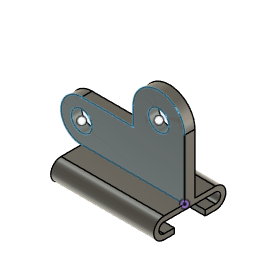
que6 v3 (Autodesk Fusion 360 design; units mm, degrees)
Autodesk Fusion 360 part; units mm, degrees
sketch "Sketch1" plane through (0, 0, 0) normal (0, 1, 0) x (1, 0, 0)
  line L0 (0, 0) -> (0, -58)
  line L1 (-50, -58) -> (-50, -40)
  line L2 (-50, -40) -> (-100, -40)
  line L3 (-100, 0) -> (0, 0)
  arc A0 (-50, -58) -> (0, -58) centre (-25, -58) ccw
  arc A1 (-100, 0) -> (-100, -40) centre (-100, -20) ccw
  circle A2 centre (-25, -58) radius 10
  circle A3 centre (-100, -20) radius 10
  dimension "d1" = 58
  dimension "d3" = 50
  dimension "d4" = 18
  dimension "d5" = 50
  dimension "d6" = 20
  dimension "d7" = 20
  constraint coincident L0.start L3.end
  constraint vertical L0
  constraint perpendicular L1 L2
  constraint concentric A0 A2
  constraint concentric A1 A3
  measures "d1" distance of L0.start L0.end
  measures "d3" distance of L0.end L1.start
  measures "d4" distance of L1.start L1.end
  measures "d5" distance of L1.end L2.end
  measures "d6" diameter of A2
  measures "d7" diameter of A3
extrude "Extrude1" add sketch "Sketch1" along normal blind 10
sketch "Sketch4" plane through (0, 0, 0) normal (1, 0, 0) x (0, 1, 0)
  line L0 (30, 0) -> (-20, 0)
  arc A0 (-20, 0) -> (-20, -20) centre (-20, -10) ccw
  line L1 (-20, -20) -> (-10, -20)
  line L2 (-10, -20) -> (-10, -15)
  line L3 (-10, -15) -> (-20, -15)
  arc A1 (-20, -5) -> (-20, -15) centre (-20, -10) ccw
  line L4 (-20, -5) -> (30, -5)
  arc A2 (30, -15) -> (30, -5) centre (30, -10) ccw
  line L5 (30, -15) -> (20, -15)
  line L6 (20, -15) -> (20, -20)
  line L7 (20, -20) -> (30, -20)
  arc A3 (30, -20) -> (30, 0) centre (30, -10) ccw
  line L8 (0, 0) -> (-20, 0)
  dimension "d24" = 50
  dimension "d25" = 5
  dimension "d26" = 10
  dimension "d28" = 5
  dimension "d29" = 5
  dimension "d31" = 10
  dimension "d32" = 5
  dimension "d33" = 5
  dimension "d34" = 10
  dimension "d35" = 20
  constraint horizontal L0
  constraint tangent L0 A0
  constraint tangent A0 L1
  constraint parallel L0 L1
  constraint perpendicular L1 L2
  constraint perpendicular L2 L3
  constraint tangent L3 A1
  constraint tangent A1 L4
  constraint parallel L3 L4
  constraint tangent L4 A2
  constraint concentric A0 A1
  constraint tangent A2 L5
  constraint horizontal L5
  constraint perpendicular L5 L6
  constraint perpendicular L6 L7
  constraint tangent L7 A3
  constraint tangent L0 A3
  constraint coincident L8.start origin
  constraint horizontal L8
  measures "d24" distance of L0.start L0.end
  measures "d25" distance of L1.end L2.end
  measures "d26" distance of L2.end L3.end
  measures "d28" distance of A0.centre L4
  measures "d29" distance of L0 L4
  measures "d31" distance of A2.start L5.end
  measures "d32" distance of L5.end L6.end
  measures "d33" radius of A2
  measures "d34" distance of L6.end L7.end
  measures "d35" distance of L8.start L0.end
extrude "Extrude2" add sketch "Sketch4" against normal blind 100
